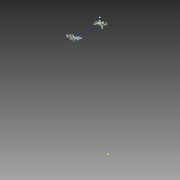
# Autodesk Inventor part: servo mount
Saved by Autodesk Inventor 2015 (Build 190159000, 159)
## iProperties
Created: 2014-11-06
Part Number: servo mount
Material: Generic
Document SubType Name: Modeling
Designer: jesse
Density: 1 g/cm^3
Appearance: Default
Author: jesse
Autodesk Inventor part; units mm, degrees
ref_plane "YZ Plane" through (0, 0, 0) normal (1, 0, 0) x (0, 1, 0)
ref_plane "Work Plane1" through (0, 0, 0) normal (0, 0, 1) x (1, 0, 0)
ref_plane "Work Plane2" through (0, 0, 0) normal (0, 0, 1) x (1, 0, 0)
sketch "Sketch2" plane through (0, 0, 0) normal (0, 0, 1) x (1, 0, 0)
  line L0 (0, 0) -> (19.05, 0) projected
  line L1 (19.05, 0) -> (19.05, 431.8) construction
  line L2 (0, 431.8) -> (19.05, 431.8) projected
  line L3 (0, 0) -> (0, 431.8) construction
  line L4 (18.5, 323.6774) -> (1.5, 323.6774) projected
  line L5 (18.5, 323.6774) -> (19.1476, 323.6774)
  line L6 (1.5, 323.6774) -> (0, 323.6774)
  line L7 (-4.8174, 323.6774) -> (23.8674, 323.6774)
  line L8 (23.8674, 323.6774) -> (23.8674, 332.1879)
  line L9 (23.8674, 332.1879) -> (-4.8174, 332.1879)
  line L10 (-4.8174, 332.1879) -> (-4.8174, 323.6774)
  line L11 (9.525, 431.8) -> (9.525, 312.4258) construction
  line L12 (9.525, 327.9326) -> (-4.8174, 327.9326) construction
  line L13 (23.8674, 327.9326) -> (9.525, 327.9326) construction
  constraints: 18 end point, 3 equal length, 3 midpoint, 3 perpendicular, 2 collinear, 2 point on line, 1 horizontal, 1 vertical
extrude "Extrusion1" add sketch "Sketch2" along normal blind 61.9125
sketch "Sketch3" plane through (-4.8174, 323.6774, 0) normal (0, -1, 0) x (1, 0, 0)
  arc A0 (8.4674, 58.3733) -> (11.1674, 58.3733) centre (9.8174, 56.7) ccw projected
  arc A1 (18.4674, 58.3733) -> (21.1674, 58.3733) centre (19.8174, 56.7) ccw projected
  arc A2 (11.1674, 7.0267) -> (8.4674, 7.0267) centre (9.8174, 8.7) ccw projected
  arc A3 (21.1674, 7.0267) -> (18.4674, 7.0267) centre (19.8174, 8.7) ccw projected
  circle A4 centre (9.8174, 8.7) radius 2.15
  circle A5 centre (19.8174, 8.7) radius 2.15
  circle A6 centre (9.8174, 56.7) radius 2.15
  circle A7 centre (19.8174, 56.7) radius 2.15
  point P0 (4.8174, 0)
  constraints: 4 centre point, 4 coincident, 4 concentric
extrude "Extrusion2" cut sketch "Sketch3" against normal through all
sketch "Sketch4" plane through (-4.8174, 332.1879, 0) normal (0, 1, 0) x (1, 0, 0)
  line L0 (4.8174, -14.2) -> (4.8174, -51.2) projected
  line L1 (6.3174, -52.7) -> (23.3174, -52.7) projected
  line L2 (24.8174, -51.2) -> (24.8174, -14.2) projected
  line L3 (23.3174, -12.7) -> (6.3174, -12.7) projected
  line L4 (4.8174, -52.7) -> (24.8174, -52.7)
  line L5 (24.8174, -52.7) -> (24.8174, -12.7)
  line L6 (24.8174, -12.7) -> (4.8174, -12.7)
  line L7 (4.8174, -12.7) -> (4.8174, -52.7)
  point P0 (4.8174, 0)
  constraints: 8 end point, 2 parallel, 1 horizontal, 1 perpendicular, 1 point on line
extrude "Extrusion3" cut sketch "Sketch4" against normal through all
sketch "Sketch6" plane through (0, 0, 0) normal (0, 0, -1) x (-1, 0, 0)
  line L0 (4.8174, 323.6774) -> (-23.8674, 323.6774) projected
  line L1 (4.8174, 332.1879) -> (4.8174, 323.6774) projected
  line L2 (-23.8674, 332.1879) -> (4.8174, 332.1879) projected
  line L3 (-23.8674, 323.6774) -> (-23.8674, 332.1879) projected
  point P0 (0, 0)
extrude "Extrusion4" add sketch "Sketch6" along normal blind 19.05
sketch "Sketch7" plane through (-4.8174, 332.1879, 61.9125) normal (0, 1, 0) x (1, 0, 0)
  line L0 (4.8174, 70.6755) -> (4.8174, 80.9625) projected
  line L1 (4.8174, 61.9125) -> (4.8174, 70.6755) projected
  line L2 (23.8674, 61.9125) -> (23.8674, 70.6755) projected
  line L3 (23.8674, 71.4375) -> (23.8674, 80.9625) projected
  line L4 (23.8674, 61.9125) -> (4.8174, 61.9125)
  line L5 (4.8174, 61.9125) -> (4.8174, 80.9625)
  line L6 (4.8174, 80.9625) -> (23.8674, 80.9625)
  line L7 (23.8674, 80.9625) -> (23.8674, 61.9125)
  constraints: 8 end point, 2 parallel, 1 horizontal, 1 perpendicular
extrude "Extrusion5" cut sketch "Sketch7" against normal through all
sketch "Sketch8" plane through (-4.8174, 332.1879, 61.9125) normal (0, 1, 0) x (1, 0, 0)
  line L0 (28.6847, 80.9625) -> (28.6847, 0) projected
  line L1 (0, 80.9625) -> (0, 0) projected
  line L2 (4.8174, 61.9125) -> (4.8174, 80.9625) projected
  line L3 (0, 80.9625) -> (4.8174, 80.9625) projected
  line L4 (0, 80.9625) -> (0, 0) projected
  line L5 (28.6847, 0) -> (0, 0) projected
  line L6 (28.6847, 80.9625) -> (28.6847, 0) projected
  line L7 (23.8674, 80.9625) -> (28.6847, 80.9625) projected
  line L8 (23.8674, 80.9625) -> (23.8674, 61.9125) projected
  line L9 (23.8674, 61.9125) -> (4.8174, 61.9125) projected
  line L10 (24.8174, 49.2125) -> (24.8174, 9.2125) projected
  line L11 (24.8174, 9.2125) -> (4.8174, 9.2125) projected
  line L12 (4.8174, 9.2125) -> (4.8174, 49.2125) projected
  line L13 (4.8174, 49.2125) -> (24.8174, 49.2125) projected
  circle A0 centre (9.8174, 5.2125) radius 2.15 projected
  circle A1 centre (9.8174, 53.2125) radius 2.15 projected
  circle A2 centre (19.8174, 53.2125) radius 2.15 projected
  circle A3 centre (19.8174, 5.2125) radius 2.15 projected
  line L14 (28.6847, 56.7746) -> (0, 56.7746)
  line L15 (28.6847, 56.7746) -> (57.3695, 56.7746) construction
  point P0 (4.8174, 61.9125)
  dimension "d10" = 180
  constraints: 4 end point, 2 point on line, 1 collinear, 1 horizontal
  measures "d10" angle of L14 L15
extrude "Extrusion6" add sketch "Sketch8" along normal blind 12.7 contours L0 L14 L1 L3 L2 L9 L8 L7
sketch "Sketch10" plane through (23.8674, 323.6774, 61.9125) normal (1, 0, 0) x (0, 0, -1)
  point P0 (61.9125, -323.6774)
sketch "Sketch11" plane through (-4.8174, 323.6774, 61.9125) normal (-1, 0, 0) x (0, 0, 1)
  line L0 (0, 0) -> (-80.9625, 0) projected
  line L1 (0, 8.5105) -> (0, 0) projected
  line L2 (-56.7746, 8.5105) -> (0, 8.5105) projected
  line L3 (-56.7746, 8.5105) -> (-56.7746, 21.2105) projected
  line L4 (-80.9625, 21.2105) -> (-56.7746, 21.2105) projected
  line L5 (-80.9625, 0) -> (-80.9625, 21.2105) projected
  circle A0 centre (-66.9806, 14.1192) radius 1.7859
  circle A1 centre (-70.7565, 7.0913) radius 1.7859
  line L6 (-66.9806, 14.1192) -> (-66.9806, 21.2105) construction
  line L7 (-70.7565, 7.0913) -> (-70.7565, 0) construction
  line L8 (-80.9625, 0) -> (0, 0) construction
  line L9 (-70.7565, 7.0913) -> (-80.9625, 7.0913) construction
  line L10 (-80.9625, 0) -> (-80.9625, 21.2105) construction
  line L11 (-66.9806, 14.1192) -> (-56.7746, 14.1192) construction
  point P0 (-61.9125, -323.6774)
  dimension "d13" = 3.5719
  dimension "d14" = 3.5719
  constraints: 8 end point, 4 point on line, 3 perpendicular, 2 centre point, 2 parallel, 1 vertical
  measures "d13" diameter of A0
  measures "d14" diameter of A1
extrude "Extrusion7" cut sketch "Sketch11" against normal through all contours A0 | A1
sketch "Sketch12" plane through (-4.8174, 332.1879, 61.9125) normal (0, 1, 0) x (1, 0, 0)
  point P0 (4.8174, 61.9125)
move faces "Move1" translate (0, 0, 31.75) faces at (4.7442, 329.3511, 61.9125)
delete faces "Delete1" heal yes whole lump no faces at (6.978, 329.3511, 57.5427) (17.143, 329.3511, 56.527)
move faces "Move2" translate (0, 0, 18.6486) faces at (6.6667, 329.3511, 52.7)
sketch "Sketch13" plane through (-4.8174, 323.6774, 93.6625) normal (0, -1, 0) x (1, 0, 0)
  line L0 (0, -88.5246) -> (0, 0) projected
  line L1 (4.8174, -22.3139) -> (0, -22.3139)
  line L2 (0, -22.3139) -> (0, -80.9198)
  line L3 (0, -80.9198) -> (4.8174, -80.9198)
  line L4 (4.8174, -80.9198) -> (4.8174, -22.3139)
  point P0 (4.8174, -93.6625)
  constraints: 8 end point, 2 parallel, 1 horizontal, 1 perpendicular, 1 point on line
extrude "Extrusion8" cut sketch "Sketch13" against normal through all
sketch "Sketch14" plane through (-4.8174, 323.6774, 93.6625) normal (0, -1, 0) x (1, 0, 0)
  line L0 (9.8174, -84.9625) -> (9.8174, -14.9173) construction
  line L1 (19.8174, -84.9625) -> (19.8174, -14.9173) construction
  circle A0 centre (19.8174, -84.9625) radius 2.15 projected
  circle A1 centre (19.8174, -84.9625) radius 2.15
  circle A2 centre (19.8174, -14.9173) radius 1.7859
  circle A3 centre (9.8174, -14.9173) radius 1.7859
  circle A4 centre (19.8174, -84.9625) radius 1.7859
  circle A5 centre (9.8174, -84.9625) radius 1.7859
  point P0 (4.8174, -93.6625)
  dimension "d29" = 3.5719
  dimension "d30" = 3.5719
  dimension "d31" = 3.5719
  dimension "d32" = 3.5719
  constraints: 5 centre point, 4 coincident, 4 end point, 2 vertical
  measures "d29" diameter of A2
  measures "d30" diameter of A3
  measures "d31" diameter of A4
  measures "d32" diameter of A5
body "Solid1"
